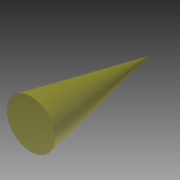
# Autodesk Inventor part: Exposure
Saved by Autodesk Inventor 2015 (Build 190159000, 159)
## iProperties
Created: 2015-03-04
Part Number: Exposure
Material: Glass
Document SubType Name: Modeling
Designer: Andrew
Density: 2.18 g/cm^3
Appearance: Clear - Yellow
Author: Andrew
Autodesk Inventor part; units mm, degrees
ref_plane "YZ Plane" through (0, 0, 0) normal (1, 0, 0) x (0, 1, 0)
ref_plane "XZ Plane" through (0, 0, 0) normal (0, 1, 0) x (-1, 0, 0)
ref_plane "XY Plane" through (0, 0, 0) normal (0, 0, 1) x (1, 0, 0)
sketch "Sketch1" plane through (0, 0, 0) normal (0, 0, 1) x (1, 0, 0)
  line L0 (0, 0) -> (40.6905, 0)
  line L1 (40.6905, 0) -> (0, 200)
  line L2 (0, 200) -> (0, 0)
  line L3 (0, 170.305) -> (6.0415, 170.305)
  dimension "d0" = 11.5
  dimension "d1" = 200
  dimension "d3" = 29.695
  constraints: 8 end point, 2 perpendicular, 2 point on line, 1 horizontal
  measures "d0" angle of L2 L1
  measures "d1" distance of L1.end L0.start
  measures "d3" distance from line of L3 L1.end
revolve "Revolution1" add sketch "Sketch1" angle 360 about axis through (0, 200, 0) along (0, -1, 0)
body "Solid1"
